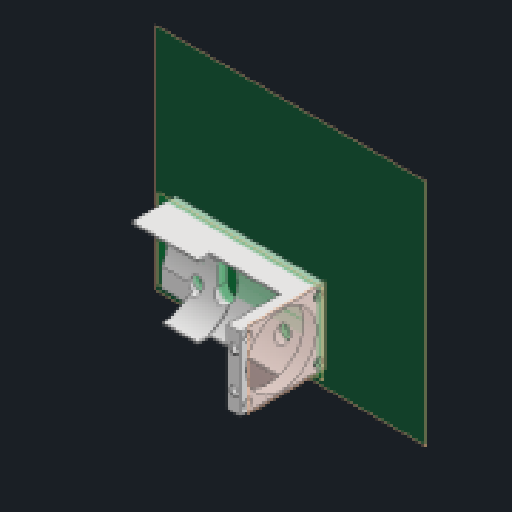
# Autodesk Inventor part: right_motor_mount
Saved by Autodesk Inventor 2023 (Build 270158000, 158)
## iProperties
Created: 2024-04-27
Part Number: right_motor_mount
Material: Generic
Document SubType Name: Modeling
Designer: szymo
Density: 1 g/cm^3
Appearance: Default
Author: szymo
Autodesk Inventor part; units mm, degrees
ref_plane "YZ Plane" through (0, 0, 0) normal (1, 0, 0) x (0, 1, 0)
ref_plane "XZ Plane" through (0, 0, 0) normal (0, 1, 0) x (-1, 0, 0)
ref_plane "XY Plane" through (0, 0, 0) normal (0, 0, 1) x (1, 0, 0)
ref_plane "Work Plane1" through (-37.7, -67.375, 15.375) normal (1, 0, 0) x (0, 0, 1)
sketch "Sketch1" plane through (-37.7, -67.375, 15.375) normal (1, 0, 0) x (0, 0, 1)
  arc A0 (7.9062, 3.651) -> (9.7035, 4.7619) centre (8.8048, 4.2064) ccw projected
  arc A1 (7.9062, 3.651) -> (4.5768, 6.4477) centre (2, 0) ccw projected
  arc A2 (5.3608, 8.4097) -> (4.5768, 6.4477) centre (4.9688, 7.4287) ccw projected
  arc A3 (9.7035, 4.7619) -> (5.3608, 8.4097) centre (2, 0) ccw projected
  arc A4 (4.5768, -6.4477) -> (5.3608, -8.4097) centre (4.9688, -7.4287) ccw projected
  arc A5 (4.5768, -6.4477) -> (7.9062, -3.651) centre (2, 0) ccw projected
  arc A6 (9.7035, -4.7619) -> (7.9062, -3.651) centre (8.8048, -4.2064) ccw projected
  arc A7 (5.3608, -8.4097) -> (9.7035, -4.7619) centre (2, 0) ccw projected
  arc A8 (-0.5553, 6.4563) -> (-1.3328, 8.4209) centre (-0.9441, 7.4386) ccw projected
  arc A9 (-0.5553, 6.4563) -> (-3.9062, 3.651) centre (2, 0) ccw projected
  arc A10 (-5.7035, 4.7619) -> (-3.9062, 3.651) centre (-4.8048, 4.2064) ccw projected
  arc A11 (-1.3328, 8.4209) -> (-5.7035, 4.7619) centre (2, 0) ccw projected
  arc A12 (-3.9062, -3.651) -> (-5.7035, -4.7619) centre (-4.8048, -4.2064) ccw projected
  arc A13 (-3.9062, -3.651) -> (-0.5553, -6.4563) centre (2, 0) ccw projected
  arc A14 (-1.3328, -8.4209) -> (-0.5553, -6.4563) centre (-0.9441, -7.4386) ccw projected
  arc A15 (-5.7035, -4.7619) -> (-1.3328, -8.4209) centre (2, 0) ccw projected
  circle A16 centre (2.0124, -10.65) radius 1.15 projected
  circle A17 centre (10, 0) radius 1.0564 projected
  circle A18 centre (-6, 0) radius 1.0564 projected
  circle A19 centre (2, 0) radius 5 projected
  circle A20 centre (2, 0) radius 13.7 projected
  line L0 (-18.375, 91.625) -> (-18.375, -14.375) projected
  line L1 (-18.375, -14.375) -> (-15.375, -14.375) projected
  line L2 (-15.375, 91.625) -> (-15.375, -14.375) projected
  line L3 (-18.375, 91.625) -> (-15.375, 91.625) projected
  circle A21 centre (2, 0) radius 14.375 projected
  line L4 (-15.375, -14.375) -> (2, -14.375)
  line L5 (2, -14.375) -> (2, 14.375)
  line L6 (2, 14.375) -> (-15.375, 14.375)
  line L7 (-15.375, 14.375) -> (-15.375, -14.375)
  line L8 (2, 14.375) -> (16.375, 14.375)
  line L9 (16.375, 14.375) -> (16.375, -14.375)
  line L10 (16.375, -14.375) -> (2, -14.375)
  line L11 (2, -14.375) -> (2, 14.375)
  point P0 (-15.375, -67.375)
  point P1 (2, 13.7)
  point P2 (-15.375, 14.375)
  point P3 (2, -13.7)
  constraints: 16 end point, 4 horizontal, 4 parallel, 2 perpendicular, 1 vertical, 1 vertical alignment, 1 other
ref_plane "Work Plane2" through (-42.7, -81.75, 1) normal (1, 0, 0) x (0, 1, 0)
extrude "Extrusion1" add sketch "Sketch1" against normal up to surface (5 mm away) contours L5 A21 A20 | L4 L2 L6 A21 picked at (-12.0468, 0.5505)
sketch "Sketch2" plane through (-42.7, -67.375, 17.375) normal (-1, 0, 0) x (0, 0, 1)
  circle A0 centre (0, 0) radius 14.375 projected
  line L0 (-17.375, 14.375) -> (-17.375, -14.375) projected
  line L1 (-17.375, -14.375) -> (0, -14.375) projected
  line L2 (0, -14.375) -> (0, -13.7) projected
  arc A1 (0, 13.7) -> (0, -13.7) centre (0, 0) ccw projected
  line L3 (0, 13.7) -> (0, 14.375) projected
  line L4 (0, 14.375) -> (-17.375, 14.375) projected
  line L5 (-17.375, 14.375) -> (0, 14.375) projected
  line L6 (-4.7286, 14.375) -> (-4.7286, 13.575)
  line L7 (0, -14.375) -> (-17.375, -14.375) projected
  line L8 (-4.7286, -14.375) -> (-4.7286, -13.575)
  point P0 (-17.375, 67.375)
  point P1 (0, -14.375)
  point P2 (0, 14.375)
  point P3 (-4.7286, -14.375)
  point P4 (-4.7286, 14.375)
  dimension "d4" = 0.8
  dimension "d5" = 0.8
  constraints: 4 end point, 2 perpendicular, 2 point on circle, 2 point on line
  measures "d4" distance of L6.start L6.end
  measures "d5" distance of L8.start L8.end
ref_plane "Work Plane3" through (-70.4, -81.75, 1) normal (-1, 0, 0) x (0, 0, 1)
extrude "Extrusion2" add sketch "Sketch2" along normal up to surface (27.7 mm away) contours A0 L8 L1 L0 L4 L6
sketch "Sketch4" plane through (-70.4, -67.375, 17.375) normal (-1, 0, 0) x (0, 0, 1)
  line L0 (-17.375, -14.375) -> (-17.375, 14.375) projected
  line L1 (-4.7286, -14.375) -> (-17.375, -14.375) projected
  arc A0 (-4.7286, 13.575) -> (-4.7286, -13.575) centre (0, 0) ccw projected
  line L2 (-17.375, 14.375) -> (-4.7286, 14.375) projected
  arc A1 (-12.9047, -4.6) -> (12.9047, -4.6) centre (0, 0) ccw projected
  line L3 (12.9047, -4.6) -> (-12.9047, -4.6) projected
  line L4 (12.9047, 4.6) -> (-12.9047, 4.6) projected
  arc A2 (12.9047, 4.6) -> (-12.9047, 4.6) centre (0, 0) ccw projected
  circle A3 centre (0, 0) radius 14.375 projected
  arc A4 (-4.7286, 13.575) -> (-4.7286, -13.575) centre (0, 0) ccw projected
  line L5 (0, -14.375) -> (0, -13.7) projected
  arc A5 (0, 13.7) -> (0, -13.7) centre (0, 0) ccw projected
  line L6 (0, 13.7) -> (0, 14.375) projected
  line L7 (-4.7286, -13.575) -> (-4.7286, -14.375) projected
  line L8 (-4.7286, -14.375) -> (0, -14.375) projected
  line L9 (0, 14.375) -> (-4.7286, 14.375) projected
  line L10 (-4.7286, 14.375) -> (-4.7286, 13.575) projected
  line L11 (-4.7286, -13.575) -> (-4.7286, -14.375) projected
  line L12 (-4.7286, 14.375) -> (-4.7286, 13.575) projected
  point P0 (-17.375, 67.375)
  point P1 (0, -14.375)
  point P2 (0, 14.375)
  point P3 (-4.7286, 14.375)
  point P4 (-4.7286, -14.375)
  point P5 (0, -13.7)
  point P6 (-12.9047, -4.6)
  point P7 (-12.9047, 4.6)
  point P8 (0, 13.7)
ref_plane "Work Plane4" through (-84.2, -81.075, 1.675) normal (-1, 0, 0) x (0, 0, 1)
extrude "Extrusion3" add sketch "Sketch4" along normal up to surface (13.8 mm away) contours L0 L2 L10 A0 L7 L1 | L7 A3 L8 | L9 A3 L10 | A0 A3 L6 A2 A5 A1 L5
sketch "Sketch5" plane through (-84.2, -67.375, 17.375) normal (-1, 0, 0) x (0, 0, 1)
  line L0 (0, 14.375) -> (0, 13.7) projected
  line L1 (-17.375, 14.375) -> (0, 14.375) projected
  line L2 (-17.375, -14.375) -> (-17.375, 14.375) projected
  line L3 (0, -14.375) -> (-17.375, -14.375) projected
  line L4 (0, -13.7) -> (0, -14.375) projected
  arc A0 (0, 13.7) -> (0, -13.7) centre (0, 0) ccw projected
  circle A1 centre (-14.625, -11.625) radius 2.75
  line L5 (-11.875, -14.375) -> (-11.875, -6.8319)
  line L6 (-11.875, -14.375) -> (-4.3319, -14.375) construction
  point P0 (-17.375, 67.375)
  dimension "d8" = 5.5
  dimension "d9" = 2.75
  dimension "d10" = 2.75
  dimension "d11" = 90
  constraints: 4 end point, 1 centre point, 1 horizontal, 1 perpendicular, 1 point on circle, 1 point on line, 1 tangent
  measures "d8" diameter of A1
  measures "d9" distance from line of A1.centre L2
  measures "d10" distance from line of A1.centre L3
  measures "d11" angle of L6 L5
ref_plane "Work Plane5" through (-96.5, -97.7889, 0) normal (1, 0, 0) x (0, 1, 0)
extrude "Extrusion4" add sketch "Sketch5" along normal up to surface (12.3 mm away) contours L0 A0 L5 A1 L2 L1 | A1 L3 L2 | A1 | L5 L3 A1
sketch "Sketch6" plane through (0, 0, 0) normal (0, 0, 1) x (1, 0, 0)
  spline S0 degree 3 poles (-70.4, -71.975) (-70.4, -72.2866) (-70.4639, -72.6146) (-70.7194, -73.215) (-70.9108, -73.4875) (-71.3398, -73.9008) (-71.6002, -74.077) (-72.1789, -74.3142) (-72.4974, -74.375) (-73.1026, -74.375) (-73.4211, -74.3142) (-73.9998, -74.077) (-74.2602, -73.9008) (-74.6892, -73.4875) (-74.8806, -73.215) (-75.1361, -72.6146) (-75.2, -72.2866) (-75.2, -71.975) knots 0.368505 0.368505 0.368505 0.368505 0.467732 0.467732 0.566959 0.566959 0.657744 0.657744 0.74853 0.74853 0.839316 0.839316 0.930102 0.930102 1.029329 1.029329 1.128556 1.128556 1.128556 1.128556 projected
  line L0 (-70.4, -53) -> (-70.4, -81.75) projected
  spline S1 degree 3 poles (-75.2, -62.775) (-75.2, -62.4634) (-75.1361, -62.1354) (-74.8806, -61.535) (-74.6892, -61.2625) (-74.2602, -60.8492) (-73.9998, -60.673) (-73.4211, -60.4358) (-73.1026, -60.375) (-72.8, -60.375) (-72.4974, -60.375) (-72.1789, -60.4358) (-71.6002, -60.673) (-71.3398, -60.8492) (-70.9108, -61.2625) (-70.7194, -61.535) (-70.4639, -62.1354) (-70.4, -62.4634) (-70.4, -62.775) knots -0.380025 -0.380025 -0.380025 -0.380025 -0.280799 -0.280799 -0.181572 -0.181572 -0.090786 -0.090786 0 0 0 0.090786 0.090786 0.181572 0.181572 0.280799 0.280799 0.380025 0.380025 0.380025 0.380025 projected
  line L1 (-75.2, -62.775) -> (-75.2, -71.975) projected
  line L2 (-76.2, -71.975) -> (-76.2, -62.775)
  line L3 (-69.4, -62.775) -> (-69.4, -71.975)
  spline S2 degree 5 poles (-69.4, -71.975) (-69.3997, -72.3257) (-69.4479, -72.6753) (-69.5344, -73.0192) (-69.803, -73.6712) (-70.2246, -74.2353) (-70.47, -74.4891) (-71.0383, -74.9353) (-71.7016, -75.2266) (-72.0624, -75.322) (-72.8, -75.4281) (-73.5376, -75.322) (-73.8984, -75.2266) (-74.5617, -74.9353) (-75.13, -74.4891) (-75.3754, -74.2353) (-75.797, -73.6712) (-76.0656, -73.0192) (-76.1521, -72.6753) (-76.2003, -72.3257) (-76.2, -71.975) knots 0 0 0 0 0 0 0.164089 0.164089 0.164089 0.32728 0.32728 0.32728 0.5 0.5 0.5 0.67272 0.67272 0.67272 0.835911 0.835911 0.835911 1 1 1 1 1 1
  spline S3 degree 5 poles (-76.2, -62.775) (-76.2003, -62.4243) (-76.1521, -62.0747) (-76.0656, -61.7308) (-75.797, -61.0788) (-75.3754, -60.5147) (-75.13, -60.2609) (-74.5617, -59.8147) (-73.8984, -59.5234) (-73.5376, -59.428) (-72.8, -59.3219) (-72.0624, -59.428) (-71.7016, -59.5234) (-71.0383, -59.8147) (-70.47, -60.2609) (-70.2246, -60.5147) (-69.803, -61.0788) (-69.5344, -61.7308) (-69.4479, -62.0747) (-69.3997, -62.4243) (-69.4, -62.775) knots 0 0 0 0 0 0 0.164089 0.164089 0.164089 0.32728 0.32728 0.32728 0.5 0.5 0.5 0.67272 0.67272 0.67272 0.835911 0.835911 0.835911 1 1 1 1 1 1
  point P0 (0, 0)
  dimension "d14" = 1
  constraints: 4 end point, 2 horizontal alignment, 2 parallel, 1 vertical, 4 other
  measures "d14" distance between parallel lines of L1 L2
extrude "Extrusion5" cut sketch "Sketch6" along normal blind 10
sketch "Sketch8" plane through (-96.5, -81.75, 0) normal (-1, 0, 0) x (0, 0, 1)
  circle A0 centre (2.75, 26) radius 2.75
  circle A1 centre (2.75, 2.75) radius 2.75
  line L0 (0, 28.75) -> (0, 0) projected
  line L1 (17.375, 28.75) -> (0, 28.75) projected
  line L2 (0, 0) -> (5.5, 0) projected
  point P0 (0, 81.75)
  dimension "d19" = 5.5
  dimension "d20" = 5.5
  constraints: 4 tangent, 2 centre point
  measures "d19" diameter of A1
  measures "d20" diameter of A0
hole "Hole1" at (-96.5, -55.75, 2.75) at (-96.5, -79, 2.75) direction (1, 0, 0) diameter 4 depth 7.75 counterbore diameter 4.6 counterbore depth 0.75
ref_plane "Work Plane6" through (-37.7, -67.375, 15.375) normal (1, 0, 0) x (0, 0, 1)
sketch "Sketch14" plane through (-37.7, -67.375, 15.375) normal (1, 0, 0) x (0, 0, 1)
  arc A0 (7.9062, 3.651) -> (9.7035, 4.7619) centre (8.8048, 4.2064) ccw projected
  arc A1 (7.9062, 3.651) -> (4.5768, 6.4477) centre (2, 0) ccw projected
  arc A2 (5.3608, 8.4097) -> (4.5768, 6.4477) centre (4.9688, 7.4287) ccw projected
  arc A3 (9.7035, 4.7619) -> (5.3608, 8.4097) centre (2, 0) ccw projected
  arc A4 (4.5768, -6.4477) -> (5.3608, -8.4097) centre (4.9688, -7.4287) ccw projected
  arc A5 (4.5768, -6.4477) -> (7.9062, -3.651) centre (2, 0) ccw projected
  arc A6 (9.7035, -4.7619) -> (7.9062, -3.651) centre (8.8048, -4.2064) ccw projected
  arc A7 (5.3608, -8.4097) -> (9.7035, -4.7619) centre (2, 0) ccw projected
  arc A8 (-0.5553, 6.4563) -> (-1.3328, 8.4209) centre (-0.9441, 7.4386) ccw projected
  arc A9 (-0.5553, 6.4563) -> (-3.9062, 3.651) centre (2, 0) ccw projected
  arc A10 (-5.7035, 4.7619) -> (-3.9062, 3.651) centre (-4.8048, 4.2064) ccw projected
  arc A11 (-1.3328, 8.4209) -> (-5.7035, 4.7619) centre (2, 0) ccw projected
  arc A12 (-3.9062, -3.651) -> (-5.7035, -4.7619) centre (-4.8048, -4.2064) ccw projected
  arc A13 (-3.9062, -3.651) -> (-0.5553, -6.4563) centre (2, 0) ccw projected
  arc A14 (-1.3328, -8.4209) -> (-0.5553, -6.4563) centre (-0.9441, -7.4386) ccw projected
  arc A15 (-5.7035, -4.7619) -> (-1.3328, -8.4209) centre (2, 0) ccw projected
  circle A16 centre (2.0124, -10.65) radius 1.15 projected
  circle A17 centre (10, 0) radius 1.0564 projected
  circle A18 centre (-6, 0) radius 1.0564 projected
  circle A19 centre (2, 0) radius 5 projected
  circle A20 centre (2, 0) radius 13.7 projected
  line L0 (2, 14.375) -> (-15.375, 14.375) projected
  line L1 (-15.375, 14.375) -> (-15.375, -14.375) projected
  line L2 (-15.375, -14.375) -> (2, -14.375) projected
  line L3 (2, -14.375) -> (2, -13.7) projected
  arc A21 (2, 13.7) -> (2, -13.7) centre (2, 0) ccw projected
  line L4 (2, 13.7) -> (2, 14.375) projected
  circle A22 centre (2, 0) radius 14.375 projected
  circle A23 centre (2, 0) radius 13.7 projected
  line L5 (2, 14.375) -> (16.375, 14.375)
  line L6 (16.375, 14.375) -> (16.375, -14.375)
  line L7 (16.375, -14.375) -> (2, -14.375)
  line L8 (2, -14.375) -> (2, 14.375)
  line L9 (18.125, 8.9145) -> (18.125, -8.7895) projected
  line L10 (16.375, -14.375) -> (18.125, -14.375)
  line L11 (18.125, -14.375) -> (18.125, 14.375)
  line L12 (18.125, 14.375) -> (16.375, 14.375)
  line L13 (16.375, 14.375) -> (16.375, -14.375)
  point P0 (-15.375, -67.375)
  point P1 (2, 13.7)
  point P2 (2, -13.7)
  point P3 (2, -14.375)
  point P4 (14.375, -5.8779)
  point P5 (14.375, 5.8779)
  point P6 (2, -13.7)
  point P7 (18.125, -8.7895)
  point P8 (18.125, 8.9145)
  point P9 (16.375, 14.375)
  constraints: 16 end point, 4 parallel, 2 horizontal, 2 perpendicular, 2 tangent
extrude "Extrusion8" add sketch "Sketch14" against normal up to surface (5 mm away) contours A20 L4 A22 L3 | A22 L6 L7 | L5 L6 A22 | L6 L12 L11 L9 L10 picked at (15.9154, -2.0824)
ref_plane "Work Plane7" through (-69.4, -67.375, 3) normal (0, 0, -1) x (-1, 0, 0)
sketch "Sketch17" plane through (-69.4, -67.375, 3) normal (0, 0, -1) x (-1, 0, 0)
  line L0 (1, -7.0083) -> (1, -13.575) projected
  line L1 (-26.7, -13.575) -> (1, -13.575) projected
  line L2 (-26.7, 13.575) -> (-26.7, -13.575) projected
  line L3 (-26.7, 13.575) -> (1, 13.575) projected
  line L4 (1, 13.575) -> (1, 7.0083) projected
  line L5 (0, 4.6) -> (0, -4.6) projected
  line L6 (-12.85, 13.575) -> (-12.85, -13.575)
  line L7 (-26.7, 0) -> (-12.85, -13.575)
  line L8 (-26.7, 0) -> (-12.85, 13.575)
  point P0 (-69.4, 67.375)
  point P1 (-19.775, 6.7875)
  point P2 (-19.775, -6.7875)
  constraints: 6 end point, 5 midpoint, 2 other
hole "Hole5" at (-49.625, -60.5875, 3) at (-49.625, -74.1625, 3) direction (0, 0, -1) diameter 3.1 end through all countersink diameter 5.5 countersink angle 90 clearance for "Countersunk Flat Head Screw ISO 2009/7046" size "M2.5" standard "ISO"
sketch "Sketch18" plane through (-69.4, -67.375, 3) normal (0, 0, -1) x (-1, 0, 0)
  circle A0 centre (-19.775, 6.7875) radius 2.75 projected
  circle A1 centre (-19.775, 6.7875) radius 1.55 projected
  circle A2 centre (-19.775, -6.7875) radius 2.75 projected
  circle A3 centre (-19.775, -6.7875) radius 1.55 projected
  point P0 (-69.4, 67.375)
extrude "Extrusion9" cut sketch "Sketch18" against normal blind 10 contours A0 | A1 | A2 | A3
ref_plane "Work Plane8" through (-76.2, -67.375, 3.675) normal (0, 0, -1) x (-1, 0, 0)
sketch "Sketch24" plane through (-76.2, -67.375, 3.675) normal (0, 0, -1) x (-1, 0, 0)
  line L0 (0, -4.6) -> (0, 4.6) projected
  line L1 (-5.8, 7.0083) -> (-5.8, 13.7) projected
  line L2 (-5.8, 13.7) -> (20.3, 13.7) projected
  line L3 (20.3, -6.8319) -> (20.3, 13.7) projected
  line L4 (8, -6.8319) -> (20.3, -6.8319) projected
  line L5 (8, -6.8319) -> (8, -13.7) projected
  line L6 (-5.8, -13.7) -> (8, -13.7) projected
  line L7 (-5.8, -13.7) -> (-5.8, -7.0083) projected
  line L8 (8, -13.7) -> (20.3, -13.7)
  line L9 (20.3, -13.7) -> (20.3, -6.8319)
  line L10 (20.3, 14.375) -> (20.3, -14.375) projected
  line L11 (20.3, 0) -> (-5.8, 13.7)
  line L12 (20.3, 13.7) -> (-5.8, 0)
  line L13 (-5.8, 0) -> (20.3, -13.7)
  line L14 (-5.8, -13.7) -> (20.3, 0)
  point P0 (-76.2, 67.375)
  point P1 (7.25, 6.85)
  point P2 (7.25, -6.85)
  constraints: 12 end point, 3 midpoint, 2 collinear, 2 parallel, 1 point on line, 2 other
hole "Hole8" at (-83.45, -60.525, 3.675) at (-83.45, -74.225, 3.675) direction (0, 0, -1) diameter 2.9 end through all countersink diameter 5.5 countersink angle 90 clearance for "Countersunk Flat Head Screw ISO 2009/7046" size "M2.5" standard "ISO"
sketch "Sketch25" plane through (-76.2, -67.375, 3.675) normal (0, 0, -1) x (-1, 0, 0)
  circle A0 centre (7.25, 6.85) radius 2.75 projected
  circle A1 centre (7.25, -6.85) radius 2.75 projected
  point P0 (-76.2, 67.375)
extrude "Extrusion11" cut sketch "Sketch25" against normal blind 10
sketch "Sketch26" plane through (-37.7, -67.375, 15.375) normal (1, 0, 0) x (0, 0, -1)
  line L0 (-18.125, -14.375) -> (15.375, -14.375) projected
  line L1 (15.375, -14.375) -> (15.375, 14.375) projected
  line L2 (15.375, 14.375) -> (-18.125, 14.375) projected
  line L3 (-18.125, 14.375) -> (-18.125, -14.375) projected
  circle A0 centre (-2, 0) radius 13.7 projected
  circle A1 centre (-15.125, -11.375) radius 1.45 projected
  circle A2 centre (-15.125, 11.375) radius 1.45 projected
  circle A3 centre (12.375, 11.375) radius 1.45 projected
  circle A4 centre (12.375, -11.375) radius 1.45 projected
  point P0 (15.375, 67.375)
  constraints: 4 coincident
hole "Hole9" at (-37.7, -78.75, 30.5) at (-37.7, -56, 30.5) at (-37.7, -56, 3) at (-37.7, -78.75, 3) direction (-1, 0, 0) diameter 3 depth 3 counterbore diameter 3.5 counterbore depth 1.4
sketch "Sketch27" plane through (-37.7, -81.75, 33.5) normal (0, 0, 1) x (1, 0, 0)
  line L0 (-5, 0) -> (-5, 28.75) projected
  line L1 (0, 0) -> (-5, 0) projected
  line L2 (0, 28.75) -> (0, 0) projected
  line L3 (0, 28.75) -> (-5, 28.75) projected
  line L4 (-1.4, 1.5) -> (-1.4, 4.5) projected
  line L5 (-3, 1.5) -> (-3, 4.5) projected
  line L6 (-1.4, 24.25) -> (-1.4, 27.25) projected
  line L7 (-3, 24.25) -> (-3, 27.25) projected
  line L8 (-5, 0) -> (-32.7, 0) projected
  line L9 (0, 4.75) -> (0, 1.25) projected
  line L10 (-5, 0) -> (0, 0)
  line L11 (0, 0) -> (0, 4.536)
  line L12 (0, 4.536) -> (-5, 4.536)
  line L13 (-5, 4.536) -> (-5, 0)
  line L14 (-5, 28.75) -> (-32.7, 28.75) projected
  line L15 (0, 28.075) -> (0, 0.675) projected
  line L16 (-5, 28.75) -> (0, 28.75)
  line L17 (0, 28.75) -> (0, 24.214)
  line L18 (0, 24.214) -> (-5, 24.214)
  line L19 (-5, 24.214) -> (-5, 28.75)
  line L20 (3, 15.4314) -> (0, 15.4314)
  line L21 (3, 13.3186) -> (0, 13.3186)
  line L22 (0, 9.875) -> (-5, 9.875)
  line L23 (-5, 9.875) -> (-5, 18.875)
  line L24 (-5, 18.875) -> (0, 18.875)
  line L25 (0, 18.875) -> (0, 9.875)
  line L26 (0, 9.875) -> (-5, 4.536)
  line L27 (-5, 9.875) -> (0, 4.536)
  line L28 (0, 18.875) -> (-5, 24.214)
  line L29 (0, 24.214) -> (-5, 18.875)
  point P0 (37.7, 81.75)
  point P1 (-2.5, 7.2055)
  point P2 (-2.5, 21.5445)
  dimension "d110" = 3.4436
  dimension "d111" = 3.4436
  dimension "d112" = 9
  constraints: 36 end point, 8 parallel, 5 horizontal, 5 point on line, 3 perpendicular, 2 midpoint, 4 other
  measures "d110" distance between parallel lines of L22 L21
  measures "d111" distance between parallel lines of L24 L20
  measures "d112" distance between parallel lines of L22 L24
hole "Hole10" at (-40.2, -74.5445, 33.5) at (-40.2, -60.2055, 33.5) direction (0, 0, -1) diameter 3 depth 3 counterbore diameter 3.5 counterbore depth 0.4
equation "\"d9\" = 0.5 * d8"
equation "\"d10\" = 0.5 * d8"
equation "\"d110\" = d111"
body "Solid1"
